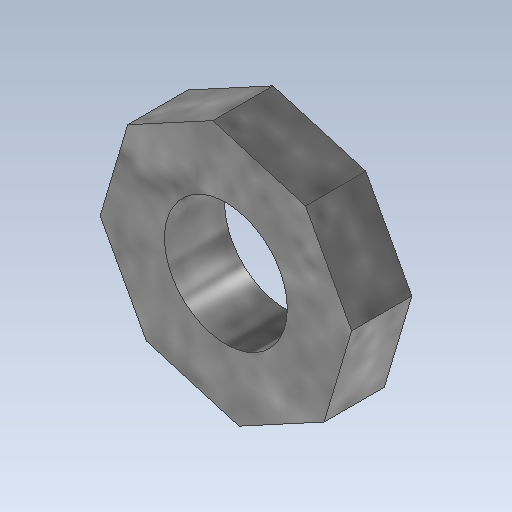
# Autodesk Inventor part: TuercaLlanta
Saved by Autodesk Inventor 2021 (Build 250183000, 183)
## iProperties
Created: 2020-12-04
Part Number: TuercaLlanta
Material: Genérico
Document SubType Name: Modeling
Designer: juanm
Density: 1 g/cm^3
Appearance: Acero galvanizado
Author: juanm
Autodesk Inventor part; units mm, degrees
ref_plane "YZ Plane" through (0, 0, 0) normal (1, 0, 0) x (0, 1, 0)
ref_plane "XZ Plane" through (0, 0, 0) normal (0, 1, 0) x (-1, 0, 0)
ref_plane "XY Plane" through (0, 0, 0) normal (0, 0, 1) x (1, 0, 0)
sketch "Boceto1" plane through (0, 0, 0) normal (0, 0, 1) x (1, 0, 0)
  circle A0 centre (0, 0) radius 10.5
  line L0 (8.1551, -6.614) -> (1.0897, -10.4433)
  line L1 (1.0897, -10.4433) -> (-6.614, -8.1551)
  line L2 (-6.614, -8.1551) -> (-10.4433, -1.0897)
  line L3 (-10.4433, -1.0897) -> (-8.1551, 6.614)
  line L4 (-8.1551, 6.614) -> (-1.0897, 10.4433)
  line L5 (-1.0897, 10.4433) -> (6.614, 8.1551)
  line L6 (6.614, 8.1551) -> (10.4433, 1.0897)
  line L7 (10.4433, 1.0897) -> (8.1551, -6.614)
  circle A1 centre (0, 0) radius 5.1
  dimension "d1" = 21
  dimension "d2" = 10.2
  constraints: 16 end point, 3 coincident, 1 centre point, 20 other
  measures "d2" diameter of A1
extrude "Extrusión1" add sketch "Boceto1" along normal blind 5 contours L7 L0 L1 L2 L3 L4 L5 L6
